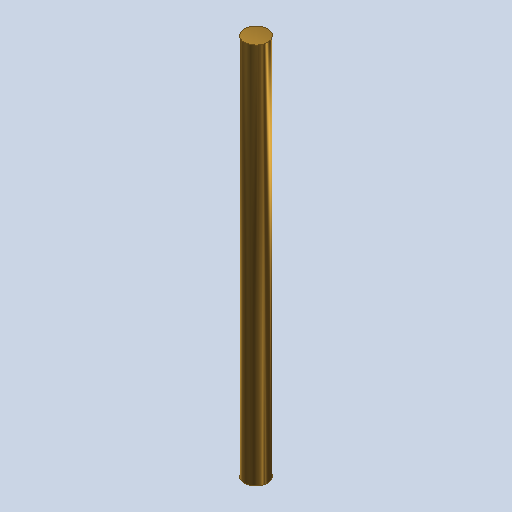
# Autodesk Inventor part: タミヤダンパー5
Saved by Autodesk Inventor 2023 (Build 270158030, 158C)
## iProperties
Part Number: タミヤダンパー5
Material: 真鍮
Document SubType Name: Modeling
Designer: 雪村
Density: 8.49 g/cm^3
Appearance: 真鍮 - つや出し
Mass: 2.9406 g
Surface Area: 4.75951 cm^2
Volume: 0.346361 cm^3
Author: 雪村
Autodesk Inventor part; units mm, degrees
ref_plane "YZ Plane" through (0, 0, 0) normal (1, 0, 0) x (0, 1, 0)
ref_plane "XZ Plane" through (0, 0, 0) normal (0, 1, 0) x (-1, 0, 0)
ref_plane "XY Plane" through (0, 0, 0) normal (0, 0, 1) x (1, 0, 0)
sketch "スケッチ1" plane through (0, 0, 0) normal (0, 0, 1) x (1, 0, 0)
  circle A0 centre (0, 0) radius 1.5
  dimension "d0" = 3
  constraints: 1 centre point, 1 coincident
  measures "d0" diameter of A0
extrude "押し出し1" add sketch "スケッチ1" along normal blind 49
